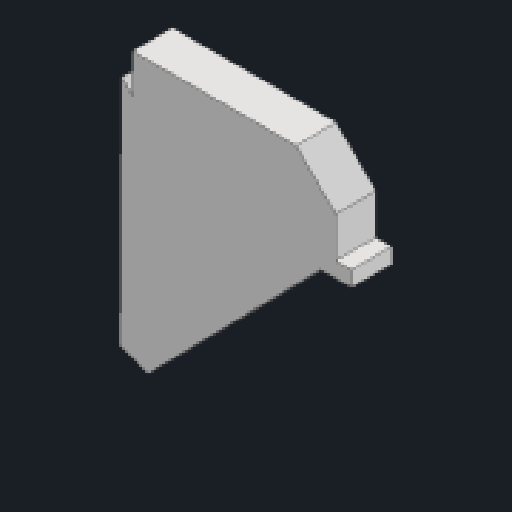
# Autodesk Inventor part: Light_guide
Saved by Autodesk Inventor 2026.2 (Build 302298000, 298)
## iProperties
Created: 2026-04-11
Part Number: Light_guide
Material: PET Plastic
Document SubType Name: Modeling
Designer: Malthe Sennels
Density: 1.541 g/cm^3
Appearance: Polycarbonate - Clear
Author: Malthe Sennels
Autodesk Inventor part; units mm, degrees
ref_plane "YZ Plane" through (0, 0, 0) normal (1, 0, 0) x (0, 1, 0)
ref_plane "XZ Plane" through (0, 0, 0) normal (0, 1, 0) x (-1, 0, 0)
ref_plane "XY Plane" through (0, 0, 0) normal (0, 0, 1) x (1, 0, 0)
sketch "Sketch1" plane through (0, 0, 0) normal (0, 0, 1) x (1, 0, 0)
  line L0 (-12.2116, 0) -> (-19.3116, 7.1)
  line L1 (-12.2116, 0) -> (7.1196, 0)
  line L2 (-15.1657, 0.0954) -> (-15.1657, 2.954)
  line L3 (-20.1702, 5.1) -> (-12.2116, -2.8586)
  line L4 (9.4454, -3) -> (-12.2116, -3)
  line L5 (0, 0) -> (0, -3)
  line L6 (-12.2116, -3) -> (-12.2116, -2.8586)
  line L7 (-15.1657, 0.0954) -> (-15.9189, 0.8486)
  line L8 (-15.9189, 0.8486) -> (-15.9189, 4.8916)
  line L9 (-15.9189, 4.8916) -> (-16.066, -16.5607)
  line L10 (-16.066, -16.5607) -> (-14.0059, -17.3004)
  line L11 (-14.0059, -17.3004) -> (0, -3)
  line L12 (-1.1297, -4.1535) -> (1.1777, -4.1535)
  line L13 (1.1777, -4.1535) -> (1.1777, -3)
  line L14 (0, -3) -> (1.1777, -3)
  line L15 (-15.1657, 2.954) -> (-2.954, 2.954)
  line L16 (-2.954, 2.954) -> (0, 0)
  point P0 (-15.9464, 0.8762)
extrude "Extrusion1" add sketch "Sketch1" along normal blind 3 contours L1 L5 L4 L6 L3 L2 L0 | L0 L15 L16 L1 | L3 L6 L4 L11 L10 L9 | L4 L13 L12 L11
body "Solid1"
